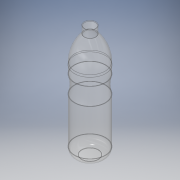
# Autodesk Inventor part: Flasche
Saved by Autodesk Inventor 2019 (Build 230136000, 136)
## iProperties
Created: 2018-09-19
Part Number: Flasche
Material: Polycarbonat, klar
Document SubType Name: Modeling
Designer: nico-
Density: 1.2 g/cm^3
Appearance: Polycarbonat - klar
Author: nico-
Autodesk Inventor part; units mm, degrees
ref_plane "YZ Plane" through (0, 0, 0) normal (1, 0, 0) x (0, 1, 0)
ref_plane "XZ Plane" through (0, 0, 0) normal (0, 1, 0) x (-1, 0, 0)
ref_plane "XY Plane" through (0, 0, 0) normal (0, 0, 1) x (1, 0, 0)
sketch "Skizze1" plane through (0, 0, 0) normal (0, 0, 1) x (1, 0, 0)
  line L0 (0, 0) -> (17, 0)
  line L1 (0, 230) -> (12, 230)
  line L2 (12, 230) -> (12, 215)
  arc A0 (32, 160) -> (12, 215) centre (-42.8985, 163.9005) ccw
  arc A1 (17, 0) -> (32, 15) centre (17, 15) ccw
  arc A2 (32, 143.7108) -> (32, 108.1134) centre (93.0349, 125.9121) ccw
  line L3 (32, 143.7108) -> (32, 160)
  line L4 (32, 108.1134) -> (32, 15)
  line L5 (0, 0) -> (0, 1)
  line L6 (0, 1) -> (17, 1)
  arc A3 (17, 1) -> (31, 15) centre (17, 15) ccw
  line L7 (31, 15) -> (31, 108.1134)
  arc A4 (31, 143.7108) -> (31, 108.1134) centre (92.5515, 125.9121) ccw
  line L8 (31, 143.7108) -> (31, 163.9005)
  arc A5 (31, 163.9005) -> (11, 214) centre (-45.2708, 162.4946) ccw
  line L9 (0, 230) -> (0, 229)
  line L10 (0, 229) -> (11, 229)
  line L11 (11, 229) -> (11, 214)
  line L12 (0, 91.5598) -> (0, 132.9573)
  point P0 (32, 0)
  dimension "d0" = 32
  dimension "d1" = 160
  dimension "d3" = 230
  dimension "d4" = 12
  dimension "d5" = 15
  dimension "d6" = 75
  dimension "d7" = 15
  dimension "d9" = 63.5771
  dimension "d17" = 93.1134
  dimension "d18" = 1
  dimension "d19" = 1
  dimension "d20" = 11
  constraints: 26 end point, 13 point on circle, 6 centre point, 6 vertical, 4 perpendicular, 3 point on line, 1 coincident, 1 horizontal, 1 parallel, 1 tangent
  measures "d0" distance of L0.start point (32, 0)
  measures "d1" distance of point (32, 0) L3.end
  measures "d3" distance of L0.start L1.start
  measures "d4" distance of L1.start L1.end
  measures "d5" distance of L1.end L2.end
  measures "d6" radius of A0
  measures "d7" radius of A1
  measures "d9" radius of A2
  measures "d17" distance of L4.start L4.end
  measures "d18" distance of L0.start L5.end
  measures "d19" distance of L1.start L9.end
  measures "d20" distance of L9.end L10.end
revolve "Umdrehung2" add sketch "Skizze1" angle 360 about axis through (0, 91.5598, 0) along (0, 1, 0)
